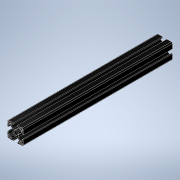
# Autodesk Inventor part: MINI-z-extrusion
Saved by Autodesk Inventor 2021 (Build 250183000, 183)
## iProperties
Created: 2019-01-15
Material: Všeobecné
Document SubType Name: Modeling
Density: 1 g/cm^3
Appearance: Hliník – tmavý
Project: ORIGINAL PRUSA MINI
Authority: Ing. Robert Turinský
Company: Prusa Development a.s.
Author: Ing. Robert Turinský
Title: MINI-z-extrusion
Revision Number: R4
Autodesk Inventor part; units mm, degrees
ref_plane "YZ Plane" through (0, 0, 0) normal (1, 0, 0) x (0, 1, 0)
ref_plane "XZ Plane" through (0, 0, 0) normal (0, 1, 0) x (-1, 0, 0)
ref_plane "XY Plane" through (0, 0, 0) normal (0, 0, 1) x (1, 0, 0)
sketch "Náčrt1" plane through (0, 0, 0) normal (0, 0, 1) x (1, 0, 0)
  line L0 (0, -21.5799) -> (0, 21.5799) projected
  line L1 (-21.5799, 0) -> (21.5799, 0) projected
  line L2 (-13, 15) -> (-4, 15)
  line L3 (-4, 15) -> (-4, 13)
  line L4 (-4, 13) -> (-8.25, 13)
  line L5 (-8.25, 13) -> (-8.25, 9.6642)
  line L6 (-8.25, 9.6642) -> (-4, 5.4142)
  line L7 (-4, 5.4142) -> (-0.5196, 5.4142)
  line L8 (-0.5196, 5.4142) -> (0, 5.1142)
  line L9 (0, 5.1142) -> (0.5196, 5.4142)
  line L10 (0.5196, 5.4142) -> (4, 5.4142)
  line L11 (4, 5.4142) -> (8.25, 9.6642)
  line L12 (8.25, 9.6642) -> (8.25, 13)
  line L13 (8.25, 13) -> (4, 13)
  line L14 (4, 13) -> (4, 15)
  line L15 (4, 15) -> (13, 15)
  line L16 (15, 13) -> (15, 4)
  line L17 (15, 4) -> (13, 4)
  line L18 (13, 4) -> (13, 8.25)
  line L19 (13, 8.25) -> (9.6642, 8.25)
  line L20 (9.6642, 8.25) -> (5.4142, 4)
  line L21 (5.4142, 4) -> (5.4142, 0.5196)
  line L22 (5.4142, 0.5196) -> (5.1142, 0)
  line L23 (5.1142, 0) -> (5.4142, -0.5196)
  line L24 (5.4142, -0.5196) -> (5.4142, -4)
  line L25 (5.4142, -4) -> (9.6642, -8.25)
  line L26 (9.6642, -8.25) -> (13, -8.25)
  line L27 (13, -8.25) -> (13, -4)
  line L28 (13, -4) -> (15, -4)
  line L29 (15, -4) -> (15, -13)
  line L30 (13, -15) -> (4, -15)
  line L31 (-15, 13) -> (-15, 4)
  line L32 (-15, 4) -> (-13, 4)
  line L33 (-13, 4) -> (-13, 8.25)
  line L34 (-13, 8.25) -> (-9.6642, 8.25)
  line L35 (-9.6642, 8.25) -> (-5.4142, 4)
  line L36 (-5.4142, 4) -> (-5.4142, 0.5196)
  line L37 (-5.4142, 0.5196) -> (-5.1142, 0)
  line L38 (-5.1142, 0) -> (-5.4142, -0.5196)
  line L39 (-5.4142, -0.5196) -> (-5.4142, -4)
  line L40 (-5.4142, -4) -> (-9.6642, -8.25)
  line L41 (-9.6642, -8.25) -> (-13, -8.25)
  line L42 (-13, -8.25) -> (-13, -4)
  line L43 (-13, -4) -> (-15, -4)
  line L44 (-15, -4) -> (-15, -13)
  line L45 (-13, -15) -> (-4, -15)
  line L46 (-4, -15) -> (-4, -13)
  line L47 (-8.25, -9.6642) -> (-4, -5.4142)
  line L48 (-4, -5.4142) -> (-0.5196, -5.4142)
  line L49 (-0.5196, -5.4142) -> (0, -5.1142)
  line L50 (0, -5.1142) -> (0.5196, -5.4142)
  line L51 (0.5196, -5.4142) -> (4, -5.4142)
  line L52 (4, -5.4142) -> (8.25, -9.6642)
  line L53 (8.25, -9.6642) -> (8.25, -13)
  line L54 (8.25, -13) -> (4, -13)
  line L55 (4, -13) -> (4, -15)
  line L56 (-4, -13) -> (-8.25, -13)
  line L57 (-8.25, -13) -> (-8.25, -9.6642)
  circle A0 centre (-11.625, 11.625) radius 2.1
  circle A1 centre (11.625, 11.625) radius 2.1
  circle A2 centre (11.625, -11.625) radius 2.1
  circle A3 centre (-11.625, -11.625) radius 2.1
  circle A4 centre (0, 0) radius 3.4
  arc A5 (-13, 15) -> (-15, 13) centre (-13, 13) ccw
  arc A6 (15, 13) -> (13, 15) centre (13, 13) ccw
  arc A7 (13, -15) -> (15, -13) centre (13, -13) ccw
  arc A8 (-15, -13) -> (-13, -15) centre (-13, -13) ccw
  line L58 (-5.1142, 0) -> (-3.4, 0)
  line L59 (0, -5.1142) -> (0, -3.4)
  line L60 (5.1142, 0) -> (3.4, 0)
  line L61 (0, 5.1142) -> (0, 3.4)
  point P0 (15, -15)
  dimension "d0" = 120
  dimension "d1" = 0.3
  dimension "d2" = 30
  dimension "d3" = 8
  dimension "d4" = 2
  dimension "d5" = 6.75
  dimension "d6" = 120
  dimension "d7" = 2
  dimension "d8" = 4.2
  dimension "d9" = 23.25
  dimension "d10" = 23.25
  dimension "d11" = 6.8
  dimension "d12" = 2
  constraints: 120 end point, 25 perpendicular, 20 point on line, 13 equal length, 12 point on circle, 9 centre point, 8 tangent, 6 parallel, 4 vertical, 3 collinear, 3 equal radius, 3 horizontal, 3 symmetric about line, 1 coincident, 37 other
  measures "d0" angle of L8 L9
  measures "d1" vertical distance of L7.end L8.end
  measures "d2" distance between parallel lines of L16 L31
  measures "d3" distance between parallel lines of L14 L3
  measures "d4" distance between parallel lines of L2 L4
  measures "d5" distance between parallel lines of L31 L5
  measures "d6" angle of L37 L38
  measures "d7" distance between parallel lines of L6 L35
  measures "d8" diameter of A0
  measures "d9" distance of A1.centre A0.centre
  measures "d10" distance of A3.centre A0.centre
  measures "d11" diameter of A4
  measures "d12" radius of A5
extrude "Vysunutí1" add sketch "Náčrt1" along normal blind 289 contours L49 L48 L47 L57 L56 L46 L45 A8 L44 L43 L42 L41 L40 L39 L38 L1 A4 L0 | L0 A4 L1 L23 L24 L25 L26 L27 L28 L29 A7 L30 L55 L54 L53 L52 L51 L50 | L1 L37 L36 L35 L34 L33 L32 L31 A5 L2 L3 L4 L5 L6 L7 L8 L0 A4 | A4 L0 L9 L10 L11 L12 L13 L14 L15 A6 L16 L17 L18 L19 L20 L21 L22 L1
thread "Závit1" size "M5x0.8" class "6H" standard "ANSI Metric M Profile" length 15
thread "Závit2" size "M4.5x0.75" class "6H" standard "ANSI Metric M Profile" length 15
thread "Závit3" size "M4.5x0.75" class "6H" standard "ANSI Metric M Profile" length 15
thread "Závit4" size "M4.5x0.75" class "6H" standard "ANSI Metric M Profile" length 15
chamfer "Zkosení1" distance 0.75 angle 45 4 edges at (9.525, 11.625, 0) (-13.725, -11.625, 0) (-13.725, -11.625, 289) (9.525, 11.625, 289)
thread "Závit5" size "M5x0.8" class "6H" standard "ANSI Metric M Profile" length 15
thread "Závit6" size "M4.5x0.75" class "6H" standard "ANSI Metric M Profile" length 15
thread "Závit7" size "M4.5x0.75" class "6H" standard "ANSI Metric M Profile" length 15
thread "Závit8" size "M4.5x0.75" class "6H" standard "ANSI Metric M Profile" length 15
chamfer "Zkosení2" distance 0.75 angle 45 4 edges at (-13.725, 11.625, 289) (9.525, -11.625, 289) (9.525, -11.625, 0) (-13.725, 11.625, 0)
chamfer "Zkosení3" distance 0.75 angle 45 2 edges at (0, -3.4, 289) (0, -3.4, 0)
equation "\"d6\" = d0"
equation "\"d7\" = d4"
